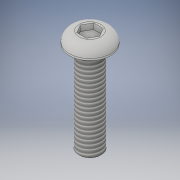
# Autodesk Inventor part: Bolt 4 mm x 16 mm
Saved by Autodesk Inventor 2018 (Build 220112000, 112)
## iProperties
Created: 2018-06-26
Part Number: Bolt 4 mm x 16 mm
Material: Generic
Document SubType Name: Modeling
Designer: Ajith Thomas
Density: 1 g/cm^3
Appearance: Default
Author: Ajith Thomas
Autodesk Inventor part; units mm, degrees
ref_plane "YZ Plane" through (0, 0, 0) normal (1, 0, 0) x (0, 1, 0)
ref_plane "XZ Plane" through (0, 0, 0) normal (0, 1, 0) x (-1, 0, 0)
ref_plane "XY Plane" through (0, 0, 0) normal (0, 0, 1) x (1, 0, 0)
sketch "Sketch1" plane through (0, 0, 0) normal (0, 1, 0) x (-1, 0, 0)
  circle A0 centre (0, 0) radius 3.6
  dimension "d0" = 7.2
  constraints: 1 centre point, 1 coincident
  measures "d0" diameter of A0
extrude "Extrusion1" add sketch "Sketch1" along normal blind 2
sketch "Sketch2" plane through (0, 2, 0) normal (0, 1, 0) x (1, 0, 0)
  line L0 (1.7034, 0) -> (0.8517, -1.4752)
  line L1 (0.8517, -1.4752) -> (-0.8517, -1.4752)
  line L2 (-0.8517, -1.4752) -> (-1.7034, 0)
  line L3 (-1.7034, 0) -> (-0.8517, 1.4752)
  line L4 (-0.8517, 1.4752) -> (0.8517, 1.4752)
  line L5 (0.8517, 1.4752) -> (1.7034, 0)
  point P0 (0, 0)
  point P1 (0, 0)
  constraints: 12 end point, 1 coincident, 13 other
extrude "Extrusion2" cut sketch "Sketch2" against normal blind 1
fillet "Fillet1" radius 1.7 1 edges at (3.6, 2, 0)
sketch "Sketch3" plane through (0, 0, 0) normal (0, -1, 0) x (1, 0, 0)
  circle A0 centre (0, 0) radius 2
  dimension "d6" = 4
  constraints: 1 centre point, 1 coincident
  measures "d6" diameter of A0
extrude "Extrusion3" add sketch "Sketch3" along normal blind 16
thread "Thread1" size "M4x0.7" class "6g" standard "ANSI Metric M Profile" full length
chamfer "Chamfer1" distance 0.2 angle 45 1 edges at (-2, -16, 0)
body "Solid1"
